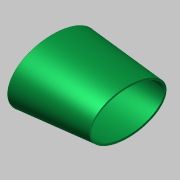
# Autodesk Inventor part: Test sweep 2012
Saved by Autodesk Inventor 2012 SP2 (Build 160200200, 200)
## iProperties
Created: 2011-05-16
Part Number: Test sweep 2012
Material: Default
Document SubType Name: Modeling
Designer: J. Lagerweij
Density: 1 g/cm^3
Author: J. Lagerweij
Autodesk Inventor part; units mm, degrees
ref_plane "YZ Plane" through (0, 0, 0) normal (1, 0, 0) x (0, 1, 0)
ref_plane "XZ Plane" through (0, 0, 0) normal (0, 1, 0) x (-1, 0, 0)
ref_plane "XY Plane" through (0, 0, 0) normal (0, 0, 1) x (1, 0, 0)
sketch "Sketch3" plane through (0, 0, 0) normal (1, 0, 0) x (0, 1, 0)
  ellipse E0 centre (0, 0) end of major axis (85, 0) minor radius 50
  point P0 (85, 0)
  dimension "d4" = 50
  constraints: 1 coincident, 1 horizontal alignment, 2 other
sketch "Sketch1" plane through (0, 0, 0) normal (0, 0, 1) x (1, 0, 0)
  line L0 (-0.3486, 81.0152) -> (-167.7093, 95.6574)
  line L1 (-167.7093, 95.6574) -> (-167.3607, 99.6422)
  line L2 (-167.3607, 99.6422) -> (0, 85)
  line L3 (0, 85) -> (-0.3486, 81.0152)
  line L4 (0, 0) -> (-15.6353, 0) construction
  dimension "d0" = 4
  dimension "d1" = 85
  dimension "d2" = 5
  dimension "d3" = 168
  constraints: 10 end point, 2 perpendicular, 1 horizontal, 1 parallel, 1 vertical alignment
  measures "d0" distance of L0.end L1.end
  measures "d1" distance of L2.end L4.start
  measures "d2" angle of L0 L4
  measures "d3" distance of L1.end L2.end
sweep "Sweep1" add profiles "Sketch1" path "Sketch3"
body "Solid1"
